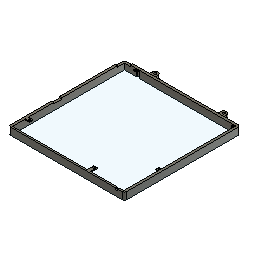
backing_plate (Autodesk Fusion 360 design; units mm, degrees)
Autodesk Fusion 360 part; units mm, degrees
sketch "Sketch1" plane through (0, 0, 0) normal (0, 1, 0) x (1, 0, 0)
  line L0 (0, 0) -> (245, 0)
  line L1 (245, 0) -> (245, -245)
  line L2 (245, -245) -> (0, -245)
  line L3 (0, -245) -> (0, 0)
  line L4 (0, 0) -> (5, 0)
  line L5 (5, 0) -> (5, -5)
  line L6 (245, -245) -> (245, -250)
  line L7 (245, -240) -> (240, -240)
  line L8 (240, -240) -> (5, -240)
  line L9 (5, -240) -> (5, -5)
  line L10 (5, -5) -> (240, -5)
  line L11 (240, -5) -> (240, -240)
  dimension "d1" = 245
  dimension "d2" = 245
  dimension "d3" = 5
  dimension "d4" = 5
  dimension "d5" = 5
  constraint horizontal L0
  constraint vertical L1
  constraint horizontal L2
  constraint vertical L3
  constraint coincident L0.start L3.end
  constraint coincident L0 L4.end
  constraint perpendicular L0 L5
  constraint coincident L1 L6.end
  constraint coincident L1 L7.start
  constraint perpendicular L1 L7
  constraint horizontal L8
  constraint vertical L9
  constraint horizontal L10
  constraint vertical L11
  measures "d1" distance of L0.start L0.end
  measures "d2" distance of L0.start L2.end
  measures "d3" distance of L0.start L4.end
  measures "d4" distance of L4.end L5.end
  measures "d5" distance of L1.end L6.end
extrude "Extrude1" add sketch "Sketch1" along normal blind 15 contours L0 L1 L2 L3 L4 L5 L7 L8 L9 | L0 L1 L5 L7 L10 L11
fillet "Fillet1" radius 5 4 edges at (0, 7.5, 0) (245, 7.5, 0) (0, 7.5, 245) (245, 7.5, 245)
sketch "Sketch2" plane through (0, 15, 0) normal (0, 1, 0) x (-1, 0, 0)
  line L0 (-5, 5) -> (-240, 5)
  line L1 (-240, 5) -> (-240, 240)
  line L2 (-240, 240) -> (-5, 240)
  line L3 (-5, 240) -> (-5, 5)
  arc A0 (-240, 245) -> (-245, 240) centre (-240, 240) ccw
  line L4 (-245, 240) -> (-245, 5)
  arc A1 (-245, 5) -> (-240, 0) centre (-240, 5) ccw
  line L5 (-240, 0) -> (-5, 0)
  arc A2 (-5, 0) -> (0, 5) centre (-5, 5) ccw
  line L6 (0, 5) -> (0, 240)
  arc A3 (0, 240) -> (-5, 245) centre (-5, 240) ccw
  line L7 (-5, 245) -> (-240, 245)
  line L8 (-245, 6.2462) -> (-238.5, 6.2462)
  line L9 (-238.7853, 0) -> (-238.7853, 6.5)
  line L10 (-238.7853, 6.5) -> (-238.5, 6.5)
  line L11 (-238.5, 6.5) -> (-238.5, 6.2462)
  circle A4 centre (-238.5, 6.5) radius 1.75
  line L12 (-20, 0) -> (-20, 6.5)
  line L13 (-20, 6.5) -> (3, 6.5)
  line L14 (0, 6.5) -> (-33, 6.5)
  circle A5 centre (-33, 6.5) radius 1.75
  line L15 (-238.5, 8.25) -> (-238.5, 9.75)
  line L16 (-238.5, 6.5) -> (-235, 6.4999)
  line L17 (-238.5, 9.75) -> (-240, 9.75)
  line L18 (-235, 6.4999) -> (-234.9999, 9.75)
  line L19 (-234.9999, 9.75) -> (-238.5, 9.75)
  line L20 (-235, 6.4999) -> (-235, 5)
  line L21 (-235, 5) -> (-240, 5)
  line L22 (-33, 6.5) -> (-33, 10)
  line L23 (-33, 6.5) -> (-36.5, 6.5)
  line L24 (-33, 6.5) -> (-36.5, 6.5)
  line L25 (-36.5, 6.5) -> (-36.5, 10)
  line L26 (-36.5, 10) -> (-33, 10)
  line L27 (-33, 10) -> (-29.5, 10)
  line L28 (-29.5, 10) -> (-29.5, 5)
  line L29 (-36.5, 6.5) -> (-36.5, 5)
  line L30 (0, 235) -> (-10.25, 235)
  line L31 (-10.25, 235) -> (-10.25, 245)
  line L32 (-10.25, 245) -> (-10.25, 210.75)
  circle A6 centre (-10.25, 210.75) radius 1.75
  line L33 (-10.25, 210.75) -> (-10.25, 207.25)
  line L34 (-10.25, 210.75) -> (-13.75, 210.75)
  line L35 (-10.25, 210.75) -> (-10.25, 207.25)
  line L36 (-10.25, 210.75) -> (-10.25, 214.25)
  line L37 (-10.25, 214.25) -> (-13.75, 214.25)
  line L38 (-13.75, 214.25) -> (-13.75, 210.75)
  line L39 (-13.75, 210.75) -> (-13.75, 207.25)
  line L40 (-13.75, 207.25) -> (-5, 207.25)
  line L41 (-10.25, 214.25) -> (-5, 214.25)
  line L42 (-198.5173, 245) -> (-198.5173, 238.5)
  line L43 (-245, 237.9591) -> (-166.4, 237.9591)
  line L44 (-166.4, 237.9591) -> (-166.4, 245)
  line L45 (-166.4, 245) -> (-166.4, 231)
  circle A7 centre (-166.4, 231) radius 1.75
  line L46 (-166.4, 231) -> (-166.4, 227.5)
  line L47 (-166.4, 227.5) -> (-162.9, 227.5)
  line L48 (-166.4, 227.5) -> (-169.9, 227.5)
  line L49 (-169.9, 227.5) -> (-169.9, 240)
  line L50 (-162.9, 227.5) -> (-162.9, 240)
  line L51 (-240, 245) -> (-240, 165)
  line L52 (-240, 165) -> (-245, 165)
  line L53 (-245, 165) -> (-238.5, 165)
  circle A8 centre (-238.5, 165) radius 1.75
  line L54 (-238.5, 165) -> (-235, 165)
  line L55 (-235, 165) -> (-235, 161.5)
  line L56 (-235, 165) -> (-235, 168.5)
  line L57 (-235, 168.5) -> (-240, 168.5)
  line L58 (-235, 161.5) -> (-240, 161.5)
  line L59 (-5, 245) -> (-5, 154)
  line L60 (-5, 154) -> (-5, 137)
  line L61 (-5, 137) -> (0, 137)
  line L62 (0, 154) -> (-5, 154)
  line L63 (0, 154) -> (0, 137)
  dimension "d9" = 6.5
  dimension "d10" = 6.5
  dimension "d11" = 3.5
  dimension "d12" = 6.5
  dimension "d13" = 33
  dimension "d14" = 3.5
  dimension "d15" = 1.5
  dimension "d16" = 3.5
  dimension "d21" = 3.5
  dimension "d22" = 3.5
  dimension "d23" = 3.5
  dimension "d24" = 3.5
  dimension "d29" = 10.25
  dimension "d30" = 34.25
  dimension "d31" = 3.5
  dimension "d32" = 3.5
  dimension "d33" = 3.5
  dimension "d34" = 3.5
  dimension "d35" = 3.5
  dimension "d36" = 3.5
  dimension "d37" = 3.5
  dimension "d40" = 6.5
  dimension "d41" = 78.6
  dimension "d42" = 14
  dimension "d43" = 3.5
  dimension "d44" = 3.5
  dimension "d45" = 3.5
  dimension "d46" = 3.5
  dimension "d49" = 80
  dimension "d50" = 6.5
  dimension "d51" = 3.5
  dimension "d52" = 3.5
  dimension "d53" = 3.5
  dimension "d54" = 3.5
  dimension "d55" = 90
  dimension "d82" = 91
  dimension "d83" = 17
  constraint coincident L4 L8.start
  constraint perpendicular L1 L8
  constraint coincident L5 L9.start
  constraint perpendicular L8 L9
  constraint perpendicular L9 L10
  constraint coincident L10.end L11.start
  constraint coincident L5 L12.start
  constraint perpendicular L0 L12
  constraint perpendicular L6 L13
  constraint coincident L6 L14.start
  constraint coincident L13 L14.start
  constraint perpendicular L3 L14
  constraint coincident L14.end A5.centre
  constraint coincident A4 L15.start
  constraint perpendicular L0 L15
  constraint perpendicular L11 L16
  constraint coincident L1 L17.end
  constraint perpendicular L1 L17
  constraint perpendicular L16 L18
  constraint perpendicular L15 L19
  constraint coincident L0 L20.end
  constraint perpendicular L0 L20
  constraint coincident L0.end L1.start
  constraint perpendicular L14 L22
  constraint perpendicular L22 L23
  constraint coincident L14 L23.end
  constraint perpendicular L23 L25
  constraint perpendicular L22 L27
  constraint coincident L0 L28.end
  constraint perpendicular L0 L28
  constraint coincident L0 L29.end
  constraint perpendicular L0 L29
  constraint coincident L6 L30.start
  constraint perpendicular L6 L30
  constraint coincident L7 L31.end
  constraint perpendicular L7 L31
  constraint perpendicular L30 L32
  constraint coincident L32.end A6.centre
  constraint coincident L32 L33.end
  constraint perpendicular L32 L34
  constraint vertical L36
  constraint perpendicular L32 L37
  constraint perpendicular L34 L39
  constraint coincident L3 L40.end
  constraint perpendicular L3 L40
  constraint coincident L3 L41.end
  constraint perpendicular L3 L41
  constraint coincident L7 L42.start
  constraint perpendicular L2 L42
  constraint coincident L4 L43.start
  constraint perpendicular L42 L43
  constraint coincident L7 L44.end
  constraint perpendicular L7 L44
  constraint perpendicular L2 L45
  constraint coincident L45.end A7.centre
  constraint parallel L45 L46
  constraint perpendicular L46 L47
  constraint perpendicular L46 L48
  constraint coincident L2 L49.end
  constraint perpendicular L2 L49
  constraint coincident L2 L50.end
  constraint perpendicular L2 L50
  constraint coincident A0.start L7.end
  constraint coincident L1 L51.end
  constraint coincident L4 L52.end
  constraint perpendicular L4 L52
  constraint perpendicular L4 L53
  constraint coincident L53.end A8.centre
  constraint perpendicular L51 L54
  constraint perpendicular L54 L55
  constraint perpendicular L54 L56
  constraint coincident L51 L57.end
  constraint coincident L1 L58.end
  constraint perpendicular L1 L58
  constraint coincident A3.end L7.start
  constraint coincident L3 L59.end
  constraint coincident L3 L60.end
  constraint coincident L6 L61.end
  constraint perpendicular L6 L61
  constraint coincident L6 L62.start
  constraint perpendicular L60 L62
  measures "d9" distance of L8.start L8.end
  measures "d10" distance of L9.start L9.end
  measures "d11" diameter of A4
  measures "d12" distance of L12.start L12.end
  measures "d13" distance of L14.start L14.end
  measures "d14" diameter of A5
  measures "d15" distance of L15.start L15.end
  measures "d16" distance of L10.end L16.end
  measures "d21" distance of L14.end L22.end
  measures "d22" distance of L14.end L23.end
  measures "d23" distance of L14.end L23.end
  measures "d24" distance of L22.end L27.end
  measures "d29" distance of L30.start L30.end
  measures "d30" distance of L31.end L32.end
  measures "d31" diameter of A6
  measures "d32" distance of L32.end L33.end
  measures "d33" distance of L32.end L34.end
  measures "d34" distance of L32.end L33.end
  measures "d35" distance of L32.end L36.end
  measures "d36" distance of L36.end L37.end
  measures "d37" distance of L34.end L39.end
  measures "d40" distance of L42.start L42.end
  measures "d41" distance of L43.start L43.end
  measures "d42" distance of L44.end L45.end
  measures "d43" diameter of A7
  measures "d44" distance of L45.end L46.end
  measures "d45" distance of L46.end L47.end
  measures "d46" distance of L46.end L48.end
  measures "d49" distance of A0.start L51.end
  measures "d50" distance of L52.end L53.end
  measures "d51" diameter of A8
  measures "d52" distance of L53.end L54.end
  measures "d53" distance of L54.end L55.end
  measures "d54" distance of L54.end L56.end
  measures "d55" angle of L56 L57
  measures "d82" distance of A3.end L59.end
  measures "d83" distance of L59.end L60.end
extrude "Extrude16" cut sketch "Sketch2" against normal blind 2.5 contours L3 L6 L60 L61 L62 L63
extrude "Extrude8" add sketch "Sketch2" against normal blind 2 contours L1 A8 L54 L55 L58 | L1 L51 A8 L54 L56 L57
extrude "Extrude7" add sketch "Sketch2" against normal blind 2 contours L2 L43 L44 L45 L49 | L43 L45 A7 L46 L48 L49 | L2 L44 L45 A7 L46 L47 L50
extrude "Extrude6" add sketch "Sketch2" against normal blind 2 contours L3 L32 A6 L33 L35 L36 L40 L41 L59 | A6 L33 L34 L35 L39 L40 | L32 A6 L34 L36 L37 L38
extrude "Extrude4" add sketch "Sketch2" against normal blind 2 contours L0 A5 L23 L24 L29 | A5 L22 L23 L24 L25 L26 | L0 L14 A5 L28 | L14 A5 L22 L27 L28
extrude "Extrude2" add sketch "Sketch2" against normal blind 2 contours L0 A4 L16 L20 L21 | L0 L8 L9 L11 A4 L16 L21 | A4 L15 L16 L18 L19 | L0 L1 L8 L9 A4 L21 | L1 L8 L9 L10 A4 L16 | L0 L1 A4 L21 | L8 L9 L10 L11 | L1 A4 L15 L17
extrude "Extrude3" cut sketch "Sketch2" against normal blind 5 contours L0 L9 A4 L21 | L0 L8 L9 L11 A4 L16 L21 | L0 L9 A4 L21 | L0 L1 L8 L9 A4 L21 | L1 L8 L9 L10 A4 L16 | L8 L9 L10 L11 | L1 L8 A4 | L1 L8 A4
extrude "Extrude5" cut sketch "Sketch2" against normal blind 5 contours L0 A5
sketch "Sketch3" plane through (0, 0, 0) normal (0, -1, 0) x (1, 0, 0)
  arc A0 (245, 240) -> (240, 245) centre (240, 240) ccw
  line L0 (240, 245) -> (5, 245)
  arc A1 (5, 245) -> (0, 240) centre (5, 240) ccw
  line L1 (0, 240) -> (0, 5)
  arc A2 (0, 5) -> (5, 0) centre (5, 5) ccw
  line L2 (5, 0) -> (240, 0)
  arc A3 (240, 0) -> (245, 5) centre (240, 5) ccw
  line L3 (245, 5) -> (245, 240)
  line L4 (240, 5) -> (5, 5)
  line L5 (5, 5) -> (5, 240)
  line L6 (5, 240) -> (240, 240)
  line L7 (240, 240) -> (240, 5)
  line L8 (240.25, 165) -> (242.25, 165)
  line L9 (242.25, 165) -> (242.25, 167.8)
  line L10 (242.25, 165) -> (242.25, 162.2)
  line L11 (242.25, 167.8) -> (240, 167.8)
  line L12 (242.25, 162.2) -> (240, 162.2)
  line L13 (240, 167.8) -> (240, 162.2)
  dimension "d58" = 2
  dimension "d59" = 2.8
  dimension "d60" = 2.8
  constraint horizontal L8
  constraint perpendicular L8 L9
  constraint perpendicular L8 L10
  constraint coincident L7 L11.end
  constraint perpendicular L7 L11
  constraint coincident L7 L12.end
  constraint perpendicular L7 L12
  measures "d58" distance of L8.start L8.end
  measures "d59" distance of L8.end L9.end
  measures "d60" distance of L8.end L10.end
extrude "Extrude10" cut sketch "Sketch3" against normal up to surface (13 mm away) contours L7 L9 L10 L11 L12 L13
extrude "Extrude9" cut sketch "Sketch2" against normal blind 10 contours L1 L52 L53 A8 | L1 L51 L52 L53 A8
sketch "Sketch4" plane through (0, 0, 0) normal (0, -1, 0) x (1, 0, 0)
  line L0 (240, 167.8) -> (242.25, 167.8)
  line L1 (242.25, 167.8) -> (242.25, 162.2)
  line L2 (242.25, 162.2) -> (240, 162.2)
  line L3 (240, 162.2) -> (240, 5)
  line L4 (240, 5) -> (5, 5)
  line L5 (5, 5) -> (5, 240)
  line L6 (5, 240) -> (240, 240)
  line L7 (240, 240) -> (240, 167.8)
  arc A0 (245, 240) -> (240, 245) centre (240, 240) ccw
  line L8 (240, 245) -> (5, 245)
  arc A1 (5, 245) -> (0, 240) centre (5, 240) ccw
  line L9 (0, 240) -> (0, 5)
  arc A2 (0, 5) -> (5, 0) centre (5, 5) ccw
  line L10 (5, 0) -> (240, 0)
  arc A3 (240, 0) -> (245, 5) centre (240, 5) ccw
  line L11 (245, 5) -> (245, 240)
  line L12 (33, 4.75) -> (33, 2.75)
  line L13 (33, 2.75) -> (35.8, 2.75)
  line L14 (33, 2.75) -> (30.2, 2.75)
  line L15 (30.2, 2.75) -> (30.2, 5)
  line L16 (35.8, 2.75) -> (35.8, 5)
  line L17 (30.2, 5) -> (35.8, 5)
  dimension "d65" = 2
  dimension "d66" = 2.8
  dimension "d67" = 2.8
  constraint vertical L12
  constraint perpendicular L12 L13
  constraint perpendicular L12 L14
  constraint coincident L4 L15.end
  constraint perpendicular L4 L15
  constraint coincident L4 L16.end
  constraint perpendicular L4 L16
  measures "d65" distance of L12.start L12.end
  measures "d66" distance of L12.end L13.end
  measures "d67" distance of L12.end L14.end
extrude "Extrude11" cut sketch "Sketch4" against normal up to surface (13 mm away) contours L4 L13 L14 L15 L16 L17
sketch "Sketch5" plane through (0, 0, 0) normal (0, -1, 0) x (1, 0, 0)
  line L0 (30.2, 2.75) -> (30.2, 5)
  line L1 (30.2, 5) -> (5, 5)
  line L2 (5, 5) -> (5, 240)
  line L3 (5, 240) -> (240, 240)
  line L4 (240, 240) -> (240, 167.8)
  line L5 (240, 167.8) -> (242.25, 167.8)
  line L6 (242.25, 167.8) -> (242.25, 162.2)
  line L7 (242.25, 162.2) -> (240, 162.2)
  line L8 (240, 162.2) -> (240, 5)
  line L9 (240, 5) -> (35.8, 5)
  line L10 (35.8, 5) -> (35.8, 2.75)
  line L11 (35.8, 2.75) -> (30.2, 2.75)
  arc A0 (245, 240) -> (240, 245) centre (240, 240) ccw
  line L12 (240, 245) -> (5, 245)
  arc A1 (5, 245) -> (0, 240) centre (5, 240) ccw
  line L13 (0, 240) -> (0, 5)
  arc A2 (0, 5) -> (5, 0) centre (5, 5) ccw
  line L14 (5, 0) -> (240, 0)
  arc A3 (240, 0) -> (245, 5) centre (240, 5) ccw
  line L15 (245, 5) -> (245, 240)
  line L16 (238.5, 4.75) -> (238.5, 2.75)
  line L17 (238.5, 2.75) -> (235.7, 2.75)
  line L18 (235.7, 2.75) -> (235.7, 5)
  line L19 (240.25, 6.5) -> (242.25, 6.5)
  line L20 (242.25, 6.5) -> (242.25, 9.3)
  line L21 (242.25, 6.5) -> (242.25, 2)
  line L22 (238.5, 2.75) -> (242.25, 2.75)
  line L23 (235.7, 5) -> (239, 5)
  line L24 (242.25, 9.3) -> (240, 9.3)
  line L25 (240, 5.8883) -> (239, 5)
  dimension "d70" = 2
  dimension "d71" = 2.8
  dimension "d72" = 2
  dimension "d73" = 2.8
  constraint perpendicular L9 L16
  constraint perpendicular L16 L17
  constraint coincident L9 L18.end
  constraint perpendicular L9 L18
  constraint perpendicular L8 L19
  constraint perpendicular L19 L20
  constraint perpendicular L19 L21
  constraint perpendicular L21 L22
  constraint coincident L9 L23.end
  constraint coincident L8 L24.end
  constraint perpendicular L8 L24
  constraint coincident L8 L25.start
  measures "d70" distance of L16.start L16.end
  measures "d71" distance of L16.end L17.end
  measures "d72" distance of L19.start L19.end
  measures "d73" distance of L19.end L20.end
extrude "Extrude12" cut sketch "Sketch5" against normal up to surface (13 mm away) contours L8 L9 L17 L18 L20 L21 L22 L23 L24 | L8 L9 L25
sketch "Sketch6" plane through (0, 0, 0) normal (-1, 0, 0) x (0, 0, 1)
  line L0 (240, 0) -> (240, 15)
  line L1 (137, 15) -> (5, 15)
  line L2 (5, 15) -> (5, 0)
  line L3 (5, 0) -> (240, 0)
  line L4 (240, 10) -> (122.5, 10)
  line L5 (122.5, 10) -> (122.5, 23)
  line L6 (122.5, 10) -> (122.5, -7.4415)
  line L7 (122.5, -7.4415) -> (-12.4248, -7.4415)
  line L8 (-12.4248, -7.4415) -> (-12.4248, 20)
  line L9 (-12.4248, 20) -> (122.5, 23)
  line L10 (154, 15) -> (154, 12.5)
  line L11 (154, 12.5) -> (137, 12.5)
  line L12 (137, 12.5) -> (137, 15)
  line L13 (240, 15) -> (154, 15)
  constraint coincident L0 L4.start
  constraint perpendicular L2 L4
  constraint perpendicular L1 L5
  constraint perpendicular L4 L6
  constraint perpendicular L6 L7
  constraint perpendicular L7 L8
extrude "Extrude14" cut 1 faces at (57.6333, 9.3333, 240) along direction (0, 0, 1) blind 1.5
sketch "Sketch7" plane through (169.9, 0, 0) normal (1, 0, 0) x (0, 0, -1)
  line L0 (-227.5, 15) -> (-241.5, 15)
  line L1 (-241.5, 15) -> (-241.5, 13)
  line L2 (-241.5, 13) -> (-227.5, 13)
  line L3 (-227.5, 13) -> (-227.5, 15)
  line L4 (-235.8167, 13) -> (-241.5, 13)
  line L5 (-241.5, 13) -> (-241.5, 9)
  line L6 (-241.5, 9) -> (-241.5, 7)
  line L7 (-241.5, 7) -> (-235.8167, 13)
  constraint coincident L2 L4.start
  constraint coincident L1.end L2.start
  constraint perpendicular L1 L4
  constraint perpendicular L4 L5
  constraint perpendicular L4 L6
extrude "Extrude15" add sketch "Sketch7" against normal blind 7 contours L2 L4 L5 L6 L7
sketch "Sketch8" plane through (0, 15, 0) normal (0, 1, 0) x (-1, 0, 0)
  line L0 (-169.9, 241.5) -> (-169.9, 227.5)
  line L1 (-169.9, 227.5) -> (-162.9, 227.5)
  line L2 (-162.9, 227.5) -> (-162.9, 241.5)
  line L3 (-162.9, 241.5) -> (-5, 241.5)
  line L4 (-5, 241.5) -> (-5, 214.25)
  line L5 (-5, 214.25) -> (-13.75, 214.25)
  line L6 (-13.75, 214.25) -> (-13.75, 207.25)
  line L7 (-13.75, 207.25) -> (-5, 207.25)
  line L8 (-5, 207.25) -> (-5, 154)
  line L9 (-5, 154) -> (0, 154)
  line L10 (0, 154) -> (0, 240)
  arc A0 (0, 240) -> (-5, 245) centre (-5, 240) ccw
  line L11 (-5, 245) -> (-240, 245)
  arc A1 (-240, 245) -> (-245, 240) centre (-240, 240) ccw
  line L12 (-245, 240) -> (-245, 5)
  arc A2 (-245, 5) -> (-240, 0) centre (-240, 5) ccw
  line L13 (-240, 0) -> (-5, 0)
  arc A3 (-5, 0) -> (0, 5) centre (-5, 5) ccw
  line L14 (0, 5) -> (0, 137)
  line L15 (0, 137) -> (-5, 137)
  line L16 (-5, 137) -> (-5, 5)
  line L17 (-5, 5) -> (-29.5, 5)
  line L18 (-29.5, 5) -> (-29.5, 10)
  line L19 (-29.5, 10) -> (-33, 10)
  line L20 (-33, 10) -> (-36.5, 10)
  line L21 (-36.5, 10) -> (-36.5, 5)
  line L22 (-36.5, 5) -> (-235, 5)
  line L23 (-235, 5) -> (-235, 6.4999)
  line L24 (-235, 6.4999) -> (-234.9999, 9.75)
  line L25 (-234.9999, 9.75) -> (-240, 9.75)
  line L26 (-240, 9.75) -> (-240, 161.5)
  line L27 (-240, 161.5) -> (-235, 161.5)
  line L28 (-235, 161.5) -> (-235, 168.5)
  line L29 (-235, 168.5) -> (-240, 168.5)
  line L30 (-240, 168.5) -> (-240, 241.5)
  line L31 (-240, 241.5) -> (-169.9, 241.5)
  circle A4 centre (-238.5, 165) radius 1.75
  circle A5 centre (-166.4, 231) radius 1.75
  circle A6 centre (-10.25, 210.75) radius 1.75
  circle A7 centre (-238.5, 6.5) radius 1.75
  circle A8 centre (-33, 6.5) radius 1.75
  line L32 (0, 5) -> (-17, 5)
  line L33 (-17, 0) -> (0, 0)
  line L34 (0, 0) -> (0, 5)
  line L35 (-17, 5) -> (-17, 0)
  dimension "d86" = 17
  constraint coincident A3.end L14.start
  constraint coincident L17 L32.end
  constraint coincident L13 L33.start
  constraint coincident L33.end L34.start
  constraint parallel L13 L33
  constraint perpendicular L13 L35
  measures "d86" distance of A3.end L32.end
extrude "Extrude17" cut sketch "Sketch8" against normal blind 2.5 contours L13 A3 L17 L32 L33 L35
sketch "Sketch9" plane through (0, 15, 0) normal (0, 1, 0) x (-1, 0, 0)
  line L0 (-5, 5) -> (0, 5)
  line L1 (0, 5) -> (0, 137)
  line L2 (0, 137) -> (-5, 137)
  line L3 (-5, 137) -> (-5, 5)
  line L4 (0, 0) -> (0, 20)
  line L5 (-5, 20) -> (0, 20)
  line L6 (-5, 20) -> (-5, 0)
  line L7 (-5, 0) -> (0, 0)
  dimension "d89" = 20
  constraint coincident L4.start L7.end
  constraint coincident L1 L4.end
  constraint coincident L3 L5.start
  constraint perpendicular L4 L5
  constraint perpendicular L5 L6
  constraint perpendicular L4 L7
  measures "d89" distance of L4.start L4.end
extrude "Extrude18" cut sketch "Sketch9" against normal blind 2.5 contours L0 L1 L3 L4 L5 L6
sketch "Sketch10" plane through (0, 0, 0) normal (0, -1, 0) x (1, 0, 0)
  line L0 (240, 241.5) -> (240, 167.8)
  line L1 (240, 167.8) -> (242.25, 167.8)
  line L2 (242.25, 167.8) -> (242.25, 162.2)
  line L3 (242.25, 162.2) -> (240, 162.2)
  line L4 (240, 162.2) -> (240, 9.3)
  line L5 (240, 9.3) -> (242.25, 9.3)
  line L6 (242.25, 9.3) -> (242.25, 2.75)
  line L7 (242.25, 2.75) -> (235.7, 2.75)
  line L8 (235.7, 2.75) -> (235.7, 5)
  line L9 (235.7, 5) -> (35.8, 5)
  line L10 (35.8, 5) -> (35.8, 2.75)
  line L11 (35.8, 2.75) -> (30.2, 2.75)
  line L12 (30.2, 2.75) -> (30.2, 5)
  line L13 (30.2, 5) -> (5, 5)
  line L14 (5, 5) -> (5, 241.5)
  line L15 (5, 241.5) -> (240, 241.5)
  arc A0 (245, 240) -> (240, 245) centre (240, 240) ccw
  line L16 (240, 245) -> (5, 245)
  arc A1 (5, 245) -> (0, 240) centre (5, 240) ccw
  line L17 (0, 240) -> (0, 5)
  arc A2 (0, 5) -> (5, 0) centre (5, 5) ccw
  line L18 (5, 0) -> (240, 0)
  arc A3 (240, 0) -> (245, 5) centre (240, 5) ccw
  line L19 (245, 5) -> (245, 240)
  line L20 (245, 0) -> (195, 0)
  line L21 (195, 0) -> (207, 0)
  line L22 (207, 0) -> (207, -3)
  line L23 (207, -3) -> (195, -3)
  line L24 (195, -3) -> (195, 0)
  line L25 (201, -3) -> (201, -9)
  circle A4 centre (201, -9) radius 2.5
  circle A5 centre (201, -9) radius 6
  line L26 (207, -3) -> (207, -9)
  line L27 (195, -3) -> (195, -9)
  dimension "d92" = 50
  dimension "d93" = 12
  dimension "d94" = 3
  dimension "d95" = 6
  dimension "d96" = 5
  constraint coincident L18 L20.end
  constraint perpendicular L6 L20
  constraint coincident L18 L21.end
  constraint perpendicular L20 L22
  constraint perpendicular L22 L23
  constraint perpendicular L21 L24
  constraint midpoint L23 L25.start
  constraint perpendicular L23 L25
  constraint coincident L25.end A4.centre
  constraint concentric A4 A5
  constraint coincident A5 L26.end
  constraint tangent A5 L26
  constraint coincident A5 L27.end
  constraint tangent A5 L27
  measures "d92" distance of L20.start L20.end
  measures "d93" distance of L20.end L21.end
  measures "d94" distance of L21.end L22.end
  measures "d95" distance of L25.start L25.end
  measures "d96" diameter of A4
extrude "Extrude19" add sketch "Sketch10" against normal blind 12 contours L18 L20 L21 L22 L23 L24 | L23 A5 L26 | L23 A5 L27 | A5
sketch "Sketch13" plane through (0, 0, 0) normal (0, -1, 0) x (1, 0, 0)
  circle A0 centre (201, -9) radius 2.5
  line L0 (240, 241.5) -> (240, 167.8)
  line L1 (240, 167.8) -> (242.25, 167.8)
  line L2 (242.25, 167.8) -> (242.25, 162.2)
  line L3 (242.25, 162.2) -> (240, 162.2)
  line L4 (240, 162.2) -> (240, 9.3)
  line L5 (240, 9.3) -> (242.25, 9.3)
  line L6 (242.25, 9.3) -> (242.25, 2.75)
  line L7 (242.25, 2.75) -> (235.7, 2.75)
  line L8 (235.7, 2.75) -> (235.7, 5)
  line L9 (235.7, 5) -> (35.8, 5)
  line L10 (35.8, 5) -> (35.8, 2.75)
  line L11 (35.8, 2.75) -> (30.2, 2.75)
  line L12 (30.2, 2.75) -> (30.2, 5)
  line L13 (30.2, 5) -> (5, 5)
  line L14 (5, 5) -> (5, 241.5)
  line L15 (5, 241.5) -> (240, 241.5)
  arc A1 (245, 240) -> (240, 245) centre (240, 240) ccw
  line L16 (240, 245) -> (5, 245)
  arc A2 (5, 245) -> (0, 240) centre (5, 240) ccw
  line L17 (0, 240) -> (0, 5)
  arc A3 (0, 5) -> (5, 0) centre (5, 5) ccw
  line L18 (5, 0) -> (195, 0)
  line L19 (195, 0) -> (195, -3)
  line L20 (195, -3) -> (195, -9)
  arc A4 (195, -9) -> (207, -9) centre (201, -9) ccw
  line L21 (207, -9) -> (207, -3)
  line L22 (207, -3) -> (207, 0)
  line L23 (207, 0) -> (240, 0)
  arc A5 (240, 0) -> (245, 5) centre (240, 5) ccw
  line L24 (245, 5) -> (245, 240)
sketch "Sketch11" plane through (0, 0, 0) normal (0, -1, 0) x (1, 0, 0)
  circle A0 centre (201, -9) radius 2.5
  line L0 (240, 241.5) -> (240, 167.8)
  line L1 (240, 167.8) -> (242.25, 167.8)
  line L2 (242.25, 167.8) -> (242.25, 162.2)
  line L3 (242.25, 162.2) -> (240, 162.2)
  line L4 (240, 162.2) -> (240, 9.3)
  line L5 (240, 9.3) -> (242.25, 9.3)
  line L6 (242.25, 9.3) -> (242.25, 2.75)
  line L7 (242.25, 2.75) -> (235.7, 2.75)
  line L8 (235.7, 2.75) -> (235.7, 5)
  line L9 (235.7, 5) -> (35.8, 5)
  line L10 (35.8, 5) -> (35.8, 2.75)
  line L11 (35.8, 2.75) -> (30.2, 2.75)
  line L12 (30.2, 2.75) -> (30.2, 5)
  line L13 (30.2, 5) -> (5, 5)
  line L14 (5, 5) -> (5, 241.5)
  line L15 (5, 241.5) -> (240, 241.5)
  arc A1 (245, 240) -> (240, 245) centre (240, 240) ccw
  line L16 (240, 245) -> (5, 245)
  arc A2 (5, 245) -> (0, 240) centre (5, 240) ccw
  line L17 (0, 240) -> (0, 5)
  arc A3 (0, 5) -> (5, 0) centre (5, 5) ccw
  line L18 (5, 0) -> (195, 0)
  line L19 (195, 0) -> (195, -3)
  line L20 (195, -3) -> (195, -9)
  arc A4 (195, -9) -> (207, -9) centre (201, -9) ccw
  line L21 (207, -9) -> (207, -3)
  line L22 (207, -3) -> (207, 0)
  line L23 (207, 0) -> (240, 0)
  arc A5 (240, 0) -> (245, 5) centre (240, 5) ccw
  line L24 (245, 5) -> (245, 240)
  line L25 (207, 0) -> (195, 0)
  constraint coincident L22.end L23.start
  constraint coincident L18.end L19.start
extrude "Extrude20" cut sketch "Sketch11" against normal blind 3 contours L19 L20 A4 L21 L22 L25
sketch "Sketch12" plane through (0, 0, 0) normal (0, -1, 0) x (1, 0, 0)
  line L0 (5, 0) -> (240, 0)
  arc A0 (240, 0) -> (245, 5) centre (240, 5) ccw
  line L1 (245, 5) -> (245, 240)
  arc A1 (245, 240) -> (240, 245) centre (240, 240) ccw
  line L2 (240, 245) -> (5, 245)
  arc A2 (5, 245) -> (0, 240) centre (5, 240) ccw
  line L3 (0, 240) -> (0, 5)
  arc A3 (0, 5) -> (5, 0) centre (5, 5) ccw
  line L4 (240, 241.5) -> (240, 167.8)
  line L5 (240, 167.8) -> (242.25, 167.8)
  line L6 (242.25, 167.8) -> (242.25, 162.2)
  line L7 (242.25, 162.2) -> (240, 162.2)
  line L8 (240, 162.2) -> (240, 9.3)
  line L9 (240, 9.3) -> (242.25, 9.3)
  line L10 (242.25, 9.3) -> (242.25, 2.75)
  line L11 (242.25, 2.75) -> (235.7, 2.75)
  line L12 (235.7, 2.75) -> (235.7, 5)
  line L13 (235.7, 5) -> (35.8, 5)
  line L14 (35.8, 5) -> (35.8, 2.75)
  line L15 (35.8, 2.75) -> (30.2, 2.75)
  line L16 (30.2, 2.75) -> (30.2, 5)
  line L17 (30.2, 5) -> (5, 5)
  line L18 (5, 5) -> (5, 241.5)
  line L19 (5, 241.5) -> (240, 241.5)
  line L20 (0, 0) -> (50, 0)
  line L21 (50, 0) -> (62, 0)
  line L22 (62, 0) -> (62, -3)
  line L23 (62, -3) -> (50, -3)
  line L24 (50, -3) -> (50, 0)
  line L25 (56, -3) -> (56, -9)
  circle A4 centre (56, -9) radius 2.5
  circle A5 centre (56, -9) radius 6
  line L26 (50, -3) -> (50, -9)
  line L27 (62, -3) -> (62, -9)
  dimension "d101" = 50
  dimension "d102" = 12
  dimension "d103" = 3
  dimension "d104" = 6
  dimension "d105" = 5
  constraint coincident L20.start origin
  constraint perpendicular L8 L20
  constraint coincident L0 L21.end
  constraint perpendicular L0 L22
  constraint perpendicular L22 L23
  constraint perpendicular L0 L24
  constraint midpoint L23 L25.start
  constraint perpendicular L23 L25
  constraint coincident L25.end A4.centre
  constraint coincident L25.start A5
  constraint coincident A5 L26.end
  constraint tangent A5 L26
  constraint coincident A5 L27.end
  constraint tangent A5 L27
  measures "d101" distance of L20.start L20.end
  measures "d102" distance of L20.end L21.end
  measures "d103" distance of L21.end L22.end
  measures "d104" distance of L25.start L25.end
  measures "d105" diameter of A4
extrude "Extrude21" add sketch "Sketch12" against normal blind 12 contours L0 L21 L22 L23 L24 | L23 A5 L26 | L23 A5 L27 | A5
sketch "Sketch14" plane through (0, 0, 0) normal (0, -1, 0) x (1, 0, 0)
  circle A0 centre (56, -9) radius 2.5
  line L0 (5, 0) -> (50, 0)
  line L1 (50, 0) -> (50, -3)
  line L2 (50, -3) -> (50, -9)
  arc A1 (50, -9) -> (62, -9) centre (56, -9) ccw
  line L3 (62, -9) -> (62, -3)
  line L4 (62, -3) -> (62, 0)
  line L5 (62, 0) -> (240, 0)
  arc A2 (240, 0) -> (245, 5) centre (240, 5) ccw
  line L6 (245, 5) -> (245, 240)
  arc A3 (245, 240) -> (240, 245) centre (240, 240) ccw
  line L7 (240, 245) -> (5, 245)
  arc A4 (5, 245) -> (0, 240) centre (5, 240) ccw
  line L8 (0, 240) -> (0, 5)
  arc A5 (0, 5) -> (5, 0) centre (5, 5) ccw
  line L9 (240, 241.5) -> (240, 167.8)
  line L10 (240, 167.8) -> (242.25, 167.8)
  line L11 (242.25, 167.8) -> (242.25, 162.2)
  line L12 (242.25, 162.2) -> (240, 162.2)
  line L13 (240, 162.2) -> (240, 9.3)
  line L14 (240, 9.3) -> (242.25, 9.3)
  line L15 (242.25, 9.3) -> (242.25, 2.75)
  line L16 (242.25, 2.75) -> (235.7, 2.75)
  line L17 (235.7, 2.75) -> (235.7, 5)
  line L18 (235.7, 5) -> (35.8, 5)
  line L19 (35.8, 5) -> (35.8, 2.75)
  line L20 (35.8, 2.75) -> (30.2, 2.75)
  line L21 (30.2, 2.75) -> (30.2, 5)
  line L22 (30.2, 5) -> (5, 5)
  line L23 (5, 5) -> (5, 241.5)
  line L24 (5, 241.5) -> (240, 241.5)
  line L25 (50, 0) -> (62, 0)
  constraint coincident L0.end L1.start
  constraint coincident L4.end L5.start
extrude "Extrude22" cut sketch "Sketch14" against normal blind 3 contours L1 L2 A1 L3 L4 L25
sketch "Sketch15" plane through (0, 0, 245) normal (0, 0, 1) x (1, 0, 0)
  line L0 (240, 0) -> (240, 15)
  line L1 (240, 15) -> (5, 15)
  line L2 (5, 15) -> (5, 0)
  line L3 (5, 0) -> (240, 0)
  line L4 (230, 15) -> (226, 15)
  line L5 (228, 15) -> (228, 13)
  circle A0 centre (228, 13) radius 2
  line L6 (226, 15) -> (226, 13)
  line L7 (230, 15) -> (230, 13)
  dimension "d110" = 4
  dimension "d111" = 2
  constraint horizontal L4
  constraint coincident L1 L4.start
  constraint midpoint L4 L5.start
  constraint perpendicular L4 L5
  constraint coincident L5.end A0.centre
  constraint coincident L5.start A0
  constraint coincident A0 L6.end
  constraint tangent A0 L6
  constraint coincident A0 L7.end
  constraint tangent A0 L7
  measures "d110" distance of L4.start L4.end
  measures "d111" distance of L5.start L5.end
extrude "Extrude23" cut sketch "Sketch15" against normal blind 8 contours L1 L4 A0 L7 | L1 L4 A0 L6 | A0
